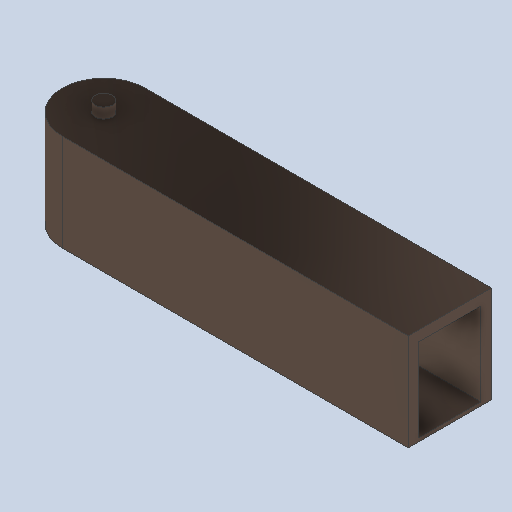
# Autodesk Inventor part: czesc2
Saved by Autodesk Inventor 2022 (Build 260153000, 153)
## iProperties
Created: 2022-06-07
Part Number: czesc2
Material: Ogólny
Document SubType Name: Sheet Metal
Designer: admin
Density: 1 g/cm^3
Sheet Metal Rule: Domyślny_mm
Appearance: Domyślna
Author: admin
Autodesk Inventor part; units mm, degrees
ref_plane "YZ Plane" through (0, 0, 0) normal (1, 0, 0) x (0, 1, 0)
ref_plane "XZ Plane" through (0, 0, 0) normal (0, 1, 0) x (-1, 0, 0)
ref_plane "XY Plane" through (0, 0, 0) normal (0, 0, 1) x (1, 0, 0)
sketch "Szkic1" plane through (0, 0, 0) normal (0, 1, 0) x (-1, 0, 0)
  circle A0 centre (0, 0) radius 60
  line L0 (0, 60) -> (-500, 60)
  line L1 (-500, 60) -> (-500, -60)
  line L2 (-500, -60) -> (0, -60)
  line L3 (0, -60) -> (0, 60)
  point P0 (0, -60)
  dimension "d0" = 120
  dimension "d1" = 500
  dimension "d2" = 120
  constraints: 8 end point, 2 horizontal, 2 parallel, 1 coincident, 1 perpendicular, 3 other
  measures "d1" distance of L2.end L1.end
  measures "d2" distance of L1.end L0.end
extrude "Wyciągnięcie proste1" add sketch "Szkic1" along normal blind 140
sketch "Szkic2" plane through (0, 140, 0) normal (0, 1, 0) x (1, 0, 0)
  circle A0 centre (0, 0) radius 12.5
  dimension "d5" = 25
  constraints: 1 centre point, 1 coincident
  measures "d5" diameter of A0
extrude "Wyciągnięcie proste2" add sketch "Szkic2" along normal blind 15
sketch "Szkic3" plane through (0, 0, 0) normal (0, -1, 0) x (1, 0, 0)
  circle A0 centre (0, 0) radius 12.5
  dimension "d8" = 25
  constraints: 1 centre point, 1 coincident
  measures "d8" diameter of A0
extrude "Wyciągnięcie proste3" add sketch "Szkic3" along normal blind 15
sketch "Szkic4" plane through (500, 0, 60) normal (1, 0, 0) x (0, 0, -1)
  line L0 (0, 0) -> (0, 140) projected
  line L1 (0, 140) -> (120, 140) projected
  line L2 (120, 0) -> (120, 140) projected
  line L3 (0, 0) -> (120, 0) projected
  line L4 (15, 125) -> (105, 125)
  line L5 (105, 125) -> (105, 5)
  line L6 (105, 5) -> (15, 5)
  line L7 (15, 5) -> (15, 125)
  line L8 (15, 125) -> (105, 5) construction
  line L9 (105, 125) -> (15, 5) construction
  point P0 (60, 0)
  point P1 (60, 65)
  dimension "d11" = 90
  dimension "d12" = 120
  dimension "d13" = 15
  dimension "d14" = 15
  constraints: 12 end point, 2 midpoint, 2 parallel, 1 horizontal, 1 perpendicular
  measures "d11" distance of L5.end L6.end
  measures "d12" distance of L4.end L5.end
  measures "d13" distance between parallel lines of L2 L5
  measures "d14" distance between parallel lines of L1 L4
extrude "Wyciągnięcie proste4" cut sketch "Szkic4" against normal blind 400 contours L4 L5 L6 L7
equation "\"PromieńGięcia\" = Grubość"
equation "\"SzerokośćGięciaPodcięcia\" = Grubość"
equation "\"GłębokośćGięciaPodcięcia\" = 0.5 * Grubość"
equation "\"RozmiarPodcięciaNarożnika\" = 4 * Grubość"
equation "\"MinimalnaPozostałość\" = 2 * Grubość"
equation "\"PromieńPrzejścia\" = PromieńGięcia"
equation "\"Rozmiar_promienia_Jacobiego\" = PromieńGięcia"
equation "\"Wielk_odstępu\" = Grubość"
equation "\"Grubość\" = 0.5"
